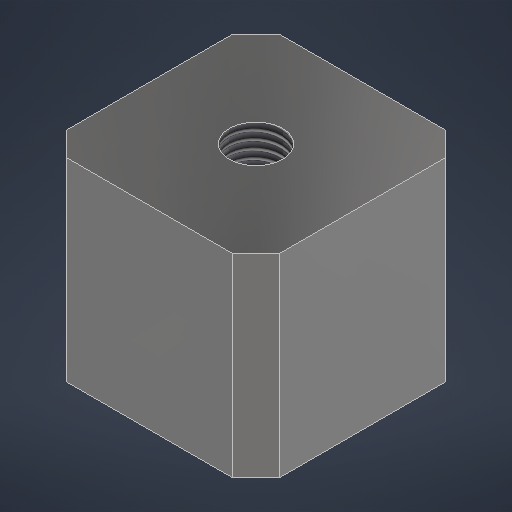
# Autodesk Inventor part: Base
Saved by Autodesk Inventor 2026 (Build 300175000, 175)
## iProperties
Created: 2025-03-21
Part Number: Base
Material: Steel, Alloy
Document SubType Name: Modeling
Designer: feder
Density: 7.73 g/cm^3
Appearance: Semi-Polished
Author: feder
Autodesk Inventor part; units mm, degrees
ref_plane "YZ Plane" through (0, 0, 0) normal (1, 0, 0) x (0, 1, 0)
ref_plane "XZ Plane" through (0, 0, 0) normal (0, 1, 0) x (-1, 0, 0)
ref_plane "XY Plane" through (0, 0, 0) normal (0, 0, 1) x (1, 0, 0)
sketch "Sketch1" plane through (0, 0, 0) normal (0, 1, 0) x (-1, 0, 0)
  line L0 (25.35, 25.35) -> (-25.35, 25.35)
  line L1 (-25.35, 25.35) -> (-25.35, -25.35)
  line L2 (-25.35, -25.35) -> (25.35, -25.35)
  line L3 (25.35, -25.35) -> (25.35, 25.35)
  line L4 (25.35, -19.6931) -> (19.6931, -25.35)
  line L5 (-19.6931, -25.35) -> (-25.35, -19.6931)
  line L6 (-25.35, 19.6931) -> (-19.6931, 25.35)
  line L7 (25.35, 19.6931) -> (19.6931, 25.35)
  point P0 (0, 0)
  point P1 (0, 25.35)
  point P2 (-25.35, 0)
  dimension "d0" = 50.7
  dimension "d1" = 50.7
  dimension "d2" = 8
  dimension "d3" = 45
  dimension "d4" = 8
  dimension "d5" = 45
  dimension "d6" = 8
  dimension "d7" = 45
  dimension "d8" = 8
  dimension "d9" = 45
  constraints: 16 end point, 8 point on line, 2 midpoint, 2 parallel, 1 horizontal, 1 horizontal alignment, 1 perpendicular, 1 vertical alignment
  measures "d0" distance of L2.end L1.end
  measures "d1" distance of L2.end L0.start
  measures "d2" distance of L4.start L4.end
  measures "d3" angle of L2 L4
  measures "d4" distance of L5.start L5.end
  measures "d5" angle of L1 L5
  measures "d6" distance of L6.start L6.end
  measures "d7" angle of L0 L6
  measures "d8" distance of L7.start L7.end
  measures "d9" angle of L7 L3
extrude "Extrusion1" add sketch "Sketch1" along normal blind 46.15 contours L7 L3 L4 L2 L5 L1 L6 L0
sketch "Sketch3" plane through (0, 46.15, 0) normal (0, 1, 0) x (1, 0, 0)
  circle A0 centre (0, 0) radius 6.35
  dimension "d13" = 12.7
  constraints: 1 centre point, 1 coincident
  measures "d13" diameter of A0
extrude "Extrusion2" cut sketch "Sketch3" against normal through all
thread "Thread3" size "1/2-13 UNC" class "2B" standard "ANSI Unified Screw Threads" length 46
body "Solid1"
